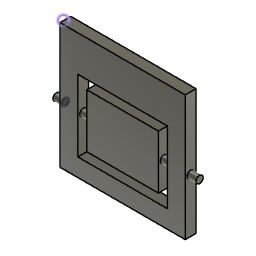
DE_Dustbin v1 (Autodesk Fusion 360 design; units mm, degrees)
Autodesk Fusion 360 part; units mm, degrees
sketch "Sketch1" plane through (0, 0, 0) normal (0, 1, 0) x (1, 0, 0)
  line L0 (0, 0) -> (35, 0)
  line L1 (35, 0) -> (35, 35)
  line L2 (35, 35) -> (0, 35)
  line L3 (0, 35) -> (0, 0)
  line L4 (5, 30) -> (30, 30)
  line L5 (30, 30) -> (30, 10)
  line L6 (30, 10) -> (5, 10)
  line L7 (5, 10) -> (5, 30)
  line L8 (7.5, 27.5) -> (27.5, 27.5)
  line L9 (27.5, 27.5) -> (27.5, 12.5)
  line L10 (27.5, 12.5) -> (7.5, 12.5)
  line L11 (7.5, 12.5) -> (7.5, 27.5)
  dimension "d1" = 35
  dimension "d2" = 35
  dimension "d3" = 10
  dimension "d4" = 5
  dimension "d5" = 30
  dimension "d6" = 30
  dimension "d19" = 12.5
  dimension "d20" = 27.5
  dimension "d21" = 7.5
  constraint coincident L0.start L3.end
  constraint horizontal L0
  constraint perpendicular L0 L1
  constraint perpendicular L1 L2
  constraint perpendicular L0 L3
  constraint horizontal L4
  constraint perpendicular L4 L5
  constraint perpendicular L5 L6
  constraint perpendicular L4 L7
  constraint perpendicular L8 L9
  constraint perpendicular L9 L10
  measures "d1" distance of L0.start L1
  measures "d2" distance of L0.start L2
  measures "d3" distance of L0.start L6
  measures "d4" distance of L0.start L7
  measures "d5" distance of L0.start L4
  measures "d6" distance of L0.start L5
  measures "d19" distance of L0.start L10
  measures "d20" distance of L0.start L8
  measures "d21" distance of L0.start L11
sketch "Sketch2" plane through (0, 0, 0) normal (0, 1, 0) x (1, 0, 0)
extrude "Extrude1" add sketch "Sketch1" along normal blind 2 contours L0 L1 L2 L3 makes body 1
extrude "Extrude2" add 1 faces at (13.3333, 0, -3.3333) along direction (0, -1, 0) blind 1 on bodies 1 bodies 1
sketch "Sketch3" plane through (0, 0, 0) normal (-1, 0, 0) x (0, -1, 0)
  line L0 (1, 0) -> (-2, 0)
  line L1 (-2, 0) -> (-2, -35)
  line L2 (-2, -35) -> (1, -35)
  line L3 (1, -35) -> (1, 0)
  circle A0 centre (-0.5, -19.9396) radius 1
  dimension "d26" = 2
  measures "d26" diameter of A0
extrude "Extrude3" cut sketch "Sketch3" against normal blind 35 contours A0 bodies 1
sketch "Sketch4" plane through (0, 2, 0) normal (0, 1, 0) x (-1, 0, 0)
  line L0 (-30, -10) -> (-5, -10)
  line L1 (-5, -10) -> (-5, -30)
  line L2 (-5, -30) -> (-30, -30)
  line L3 (-30, -30) -> (-30, -10)
  line L4 (0, -35) -> (0, 0)
  line L5 (0, 0) -> (-35, 0)
  line L6 (-35, 0) -> (-35, -35)
  line L7 (-35, -35) -> (0, -35)
  line L8 (15, -10) -> (35, -10)
  line L9 (35, -10) -> (35, -25)
  line L10 (35, -25) -> (15, -25)
  line L11 (15, -25) -> (15, -10)
  dimension "d29" = 15
  dimension "d30" = 10
  dimension "d31" = 25
  dimension "d32" = 35
  constraint horizontal L8
  constraint perpendicular L8 L9
  constraint perpendicular L9 L10
  constraint perpendicular L8 L11
  measures "d29" distance of L4.end L11
  measures "d30" distance of L4.end L8
  measures "d31" distance of L4.end L10
  measures "d32" distance of L4.end L9
sketch "Sketch5" plane through (0, 2, 0) normal (0, 1, 0) x (-1, 0, 0)
extrude "Extrude4" add sketch "Sketch4" against normal blind 3 separate body contours L8 L9 L10 L11 makes body 2
sketch "Sketch6" plane through (0, 0, 0) normal (0, 1, 0) x (1, 0, 0)
move_face "MoveFace1" by (-6.1171, 0, 20.2675) 1 faces at (-21.6667, -1, -20) on bodies 2
move_face "MoveFace2" by (0, 0, 23) 1 faces at (-21.6667, -1, -20) on bodies 2
move_body "Move1" bodies 2 to x (1, 0, 0) y (0, 1, 0) z (0, 0, 1) at (35, 0, 31)
sketch "Sketch7" plane through (0, 0, 0) normal (1, 0, 0) x (0, 1, 0)
move_body "Move2" bodies 2 to x (1, 0, 0) y (0, 1, 0) z (0, 0, 1) at (0, 0, -6)
sketch "Sketch8" plane through (0, 0, 0) normal (1, 0, 0) x (0, 1, 0)
sketch "Sketch9" plane through (0, 0, 0) normal (1, 0, 0) x (0, 1, 0)
  circle A0 centre (0.5, 7.5) radius 1
  point P0 (0.5, 7.5)
  dimension "d37" = 2
  constraint coincident P0 A0.centre
  measures "d37" diameter of A0
extrude "Extrude5" cut sketch "Sketch9" along normal blind 20 bodies 2
move_body "Move3" bodies 2 to x (1, 0, 0) y (0, 1, 0) z (0, 0, 1) at (7.5, 0, -27.5)
sketch "Sketch10" plane through (0, 0, 0) normal (1, 0, 0) x (0, 1, 0)
sketch "Sketch11" plane through (0, 0, 0) normal (-1, 0, 0) x (0, -1, 0)
  circle A0 centre (-0.5, -19.9396) radius 1
  line L0 (1, 0) -> (-2, 0)
  line L1 (-2, 0) -> (-2, -35)
  line L2 (-2, -35) -> (1, -35)
  line L3 (1, -35) -> (1, 0)
  circle A1 centre (-0.5, -19.9396) radius 1
  dimension "d41" = 2
  constraint concentric A0 A1
  measures "d41" diameter of A1
sketch "Sketch12" plane through (0, 0, 0) normal (-1, 0, 0) x (0, -1, 0)
  circle A0 centre (-0.5, -19.9396) radius 1
  point P0 (-0.5, -19.9396)
  dimension "d42" = 2
  constraint coincident P0 A0.centre
  measures "d42" diameter of A0
extrude "Extrude6" add sketch "Sketch12" against normal blind 40 separate body makes body 3
move_body "Move4" bodies 3 to x (1, 0, 0) y (0, 1, 0) z (0, 0, 1) at (-2.5, 0, 0)
copy_body "Body->Comp1" bodies 1 removing the originals makes body 4 in component "Component"
copy_body "Body->Comp2" bodies 2 removing the originals makes body 5 in component "Component'"
copy_body "Body->Comp3" bodies 3 removing the originals makes body 6 in component "Component''"
component "Component" placed x (1, 0, 0) y (0, 1, 0) z (0, 0, 1) at (0, 0, 0)
component "Component'" placed x (1, 0, 0) y (0, 1, 0) z (0, 0, 1) at (0, 0, 0)
component "Component''" placed x (1, 0, 0) y (0, 1, 0) z (0, 0, 1) at (0, 0, 0)
